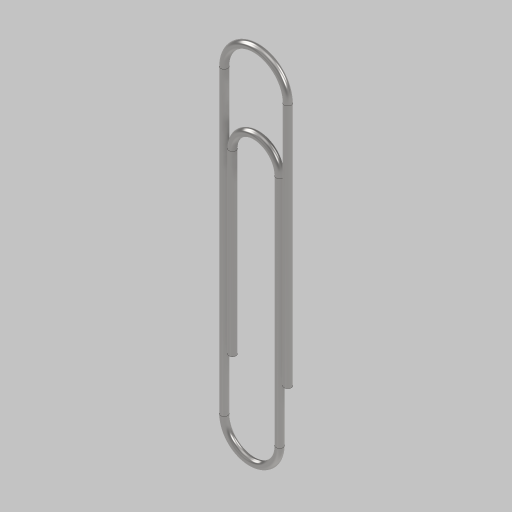
# Autodesk Inventor part: paperclip_big
Saved by Autodesk Inventor 2023.2 (Build 272271030, 271C)
## iProperties
Created: 2023-04-30
Part Number: paperclip_big
Material: Stainless Steel
Document SubType Name: Modeling
Designer: Nebojsa
Density: 8 g/cm^3
Appearance: Semi-Polished
Mass: 3.65616 g
Surface Area: 12.2226 cm^2
Volume: 0.45702 cm^3
Author: Nebojsa
Autodesk Inventor part; units mm, degrees
ref_plane "YZ Plane" through (0, 0, 0) normal (1, 0, 0) x (0, 1, 0)
ref_plane "XY Plane" through (0, 0, 0) normal (0, 0, 1) x (1, 0, 0)
sketch "Sketch1" plane through (0, 0, 0) normal (0, 0, 1) x (1, 0, 0)
  line L0 (-6.75, -38.25) -> (6.75, -38.25) construction
  line L1 (6.75, -38.25) -> (6.75, 38.25) construction
  line L2 (6.75, 38.25) -> (-6.75, 38.25) construction
  line L3 (-6.75, 38.25) -> (-6.75, -38.25) construction
  line L4 (-6.75, -38.25) -> (6.75, 38.25) construction
  line L5 (6.75, -38.25) -> (-6.75, 38.25) construction
  arc A0 (6.75, 31.5) -> (-6.75, 31.5) centre (0, 31.5) ccw
  line L6 (-6.75, 22.25) -> (6.75, 22.25) construction
  arc A1 (-6.75, -32.375) -> (5, -32.375) centre (-0.875, -32.375) ccw
  line L7 (-6.75, 31.5) -> (-6.75, -32.375)
  line L8 (6.75, 31.5) -> (6.75, -20.5)
  line L9 (5, -32.375) -> (5, 17.25)
  arc A2 (5, 17.25) -> (-5, 17.25) centre (0, 17.25) ccw
  line L10 (6.75, -20.5) -> (-6.75, -20.5) construction
  line L11 (-5, 17.25) -> (-5, -20.5)
  line L12 (0, 31.5) -> (0, -46.328) construction
  point P0 (0, 0)
  dimension "d0" = 76.5
  dimension "d1" = 13.5
  dimension "d3" = 60.5
  dimension "d5" = 52
  dimension "d11" = 1.75
  dimension "d13" = 1.75
  dimension "d14" = 1.75
  constraints: 26 end point, 10 tangent, 7 point on line, 6 point on circle, 3 centre point, 3 perpendicular, 3 vertical, 2 horizontal, 2 midpoint, 2 parallel
  measures "d0" distance of L2.end L0.start
  measures "d1" distance of L1.end L2.end
  measures "d3" distance between parallel lines of L0 L6
  measures "d5" distance of L8.start L8.end
  measures "d11" distance between parallel lines of L1 L9
  measures "d13" distance between parallel lines of L8 L9
  measures "d14" distance between parallel lines of L11 L7
ref_plane "Work Plane1" through (-5, -20.5, 0) normal (0, 1, 0) x (-1, 0, 0)
sketch "Sketch2" plane through (-5, -20.5, 0) normal (0, 1, 0) x (-1, 0, 0)
  circle A0 centre (0, 0) radius 0.75
  point P0 (-5, 0)
  dimension "d7" = 1.5
  constraints: 1 centre point, 1 coincident
  measures "d7" diameter of A0
sweep "Sweep1" add profiles "Sketch2" path "Sketch1"
equation "\"d14\" = d13"
body "Solid1"
